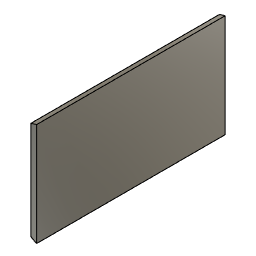
front2-top v4 (Autodesk Fusion 360 design; units mm, degrees)
Autodesk Fusion 360 part; units mm, degrees
note: some values were not read from the file. Set by a fixed rule: which sketch regions a step uses.
sketch "Esquisse1" plane through (0, 0, 0) normal (0, 1, 0) x (1, 0, 0)
  line L0 (0, -70.8995) -> (0, -2.1403)
  line L1 (4, -72.111) -> (4, 0)
  line L2 (0, -2.1403) -> (4, 0)
  line L3 (4, -72.111) -> (0, -70.8995)
  dimension "d3" = 61.85
  dimension "d6" = 72.111
  dimension "d7" = 73.15
  constraint vertical L0
  measures "d3" angle of L1 L2
  measures "d6" distance of L1.start L1.end
  measures "d7" angle of L1 L3
extrude "Extrusion1" add sketch "Esquisse1" along normal blind 132
